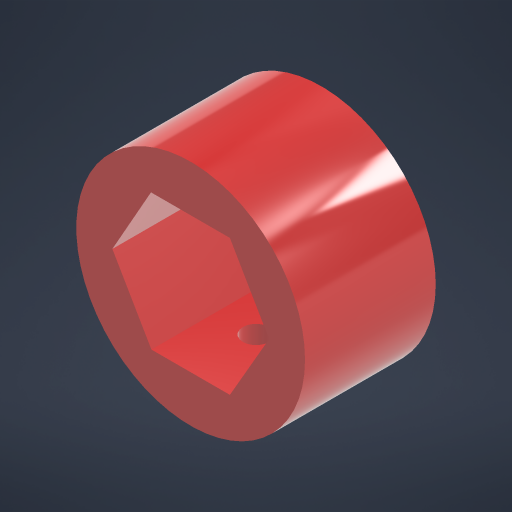
# Autodesk Inventor part: Churro Spacer
Saved by Autodesk Inventor 2024.2 (Build 282272000, 272)
## iProperties
Created: 2022-09-22
Part Number: Churro Spacer
Material: Generic
Document SubType Name: Modeling
Designer: Jason
Density: 1 g/cm^3
Appearance: Violet
Author: Jason
Autodesk Inventor part; units mm, degrees
ref_plane "YZ Plane" through (0, 0, 0) normal (1, 0, 0) x (0, 1, 0)
ref_plane "XZ Plane" through (0, 0, 0) normal (0, 1, 0) x (-1, 0, 0)
ref_plane "XY Plane" through (0, 0, 0) normal (0, 0, 1) x (1, 0, 0)
sketch "Sketch1" plane through (0, 0, 0) normal (0, 0, 1) x (1, 0, 0)
  circle A0 centre (0, 0) radius 11.1125
  line L0 (0, 0) -> (7.6256, 0)
  line L1 (-3.8526, 6.604) -> (3.8128, 6.604)
  line L2 (3.8128, 6.604) -> (7.6256, 0)
  line L3 (7.6256, 0) -> (3.8128, -6.604)
  line L4 (3.8128, -6.604) -> (-3.8128, -6.604)
  line L5 (-3.8128, -6.604) -> (-7.6056, -0.0348)
  line L6 (-7.6056, -0.0348) -> (-3.8526, 6.604)
  line L7 (0, 0) -> (0, 6.604)
  line L8 (0, 0) -> (0, -6.604)
  line L9 (0, 0) -> (-5.7192, 3.302)
  line L10 (0, 0) -> (5.7192, -3.302)
  line L11 (0, 0) -> (5.7192, 3.302)
  line L12 (0, 0) -> (-5.7192, -3.302)
  line L13 (-7.2737, 0.1016) -> (-3.7248, 6.2484)
  line L14 (-3.5489, 6.35) -> (3.5489, 6.35)
  arc A1 (3.7248, 6.2484) -> (3.5489, 6.35) centre (3.5489, 6.1468) ccw
  line L15 (3.7248, 6.2484) -> (7.2737, 0.1016)
  arc A2 (-3.5489, 6.35) -> (-3.7248, 6.2484) centre (-3.5489, 6.1468) ccw
  arc A3 (-7.2737, 0.1016) -> (-7.2737, -0.1016) centre (-7.0977, 0) ccw
  line L16 (-3.7248, -6.2484) -> (-7.2737, -0.1016)
  line L17 (3.5489, -6.35) -> (-3.5489, -6.35)
  arc A4 (-3.7248, -6.2484) -> (-3.5489, -6.35) centre (-3.5489, -6.1468) ccw
  arc A5 (3.5489, -6.35) -> (3.7248, -6.2484) centre (3.5489, -6.1468) ccw
  line L18 (7.2737, -0.1016) -> (3.7248, -6.2484)
  arc A6 (7.2737, -0.1016) -> (7.2737, 0.1016) centre (7.0977, 0) ccw
  point P0 (0, 0)
  dimension "d0" = 22.225
  dimension "d19" = 6.604
  dimension "d20" = 6.604
  dimension "d21" = 6.604
  dimension "d22" = 6.604
  dimension "d23" = 60
  dimension "d24" = 60
  dimension "d25" = 6.604
  dimension "d26" = 6.604
  dimension "d27" = 60
  dimension "d28" = 60
  dimension "d30" = 13.208
  constraints: 38 end point, 12 point on circle, 7 centre point, 3 midpoint, 2 point on line, 2 vertical, 1 coincident, 1 horizontal, 1 parallel, 1 perpendicular
  measures "d0" diameter of A0
  measures "d19" distance of L0.start L7.end
  measures "d20" distance of L0.start L8.end
  measures "d21" distance of L0.start L9.end
  measures "d22" distance of L0.start L10.end
  measures "d23" angle of L7 L9
  measures "d24" angle of L8 L10
  measures "d25" distance of L0.start L11.end
  measures "d26" distance of L0.start L12.end
  measures "d27" angle of L8 L12
  measures "d28" angle of L7 L11
  measures "d30" distance between parallel lines of L4 L1
extrude "Extrusion1" add sketch "Sketch1" along normal blind 12.7
sketch "Sketch3" plane through (-3.8128, -6.604, 0) normal (0, 1, 0) x (1, 0, 0)
  line L0 (11.4385, -12.7) -> (7.6256, -12.7) projected
  line L1 (7.6256, 0) -> (0, 0) projected
  line L2 (7.6256, -12.7) -> (0, 0)
  line L3 (7.6256, 0) -> (7.6256, -12.7) projected
  line L4 (0, 0) -> (7.6256, 0)
  line L5 (7.6256, 0) -> (7.6256, -12.7)
  line L6 (7.6256, -12.7) -> (0, -12.7) projected
  line L7 (7.6256, -12.7) -> (0, -12.7)
  line L8 (0, -12.7) -> (7.6256, 0)
  line L9 (0, 0) -> (0, -12.7)
  circle A0 centre (3.8128, -6.35) radius 1.27
  point P0 (3.8128, 0)
  dimension "d31" = 2.54
  constraints: 12 end point, 3 perpendicular, 1 centre point, 1 collinear, 1 midpoint
  measures "d31" diameter of A0
extrude "Extrusion2" cut sketch "Sketch3" against normal through all contours A0 L2 L8 | L8 L2 A0 | L2 L8 A0 | A0 L8 L2
body "Solid1"
